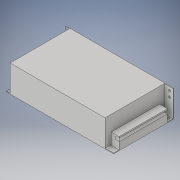
# Autodesk Inventor part: PowerS
Saved by Autodesk Inventor 2019.3 (Build 233278000, 278)
## iProperties
Created: 2020-08-28
Part Number: PowerS
Material: Generisch
Document SubType Name: Modeling
Designer: Nicolas Frick
Density: 1 g/cm^3
Appearance: Vorgabe
Author: Nicolas Frick
Autodesk Inventor part; units mm, degrees
ref_plane "YZ Plane" through (0, 0, 0) normal (1, 0, 0) x (0, 1, 0)
ref_plane "XZ Plane" through (0, 0, 0) normal (0, 1, 0) x (-1, 0, 0)
ref_plane "XY Plane" through (0, 0, 0) normal (0, 0, 1) x (1, 0, 0)
sketch "Skizze1" plane through (0, 0, 0) normal (0, 1, 0) x (-1, 0, 0)
  line L0 (88, 55) -> (-88, 55)
  line L1 (-88, 55) -> (-88, -55)
  line L2 (-88, -55) -> (88, -55)
  line L3 (88, -55) -> (88, 55)
  line L4 (88, 55) -> (-88, -55) construction
  line L5 (-88, 55) -> (88, -55) construction
  point P0 (0, 0)
  dimension "d0" = 176
  dimension "d1" = 110
  constraints: 12 end point, 2 midpoint, 2 parallel, 1 horizontal, 1 perpendicular
  measures "d0" distance of L2.end L1.end
  measures "d1" distance of L1.end L0.end
extrude "Extrusion1" add sketch "Skizze1" along normal blind 48.5
sketch "Skizze2" plane through (0, 0, 0) normal (0, -1, 0) x (1, 0, 0)
  line L0 (-88, 55) -> (88, 55) projected
  line L1 (-88, 55) -> (-95, 55)
  line L2 (-95, 55) -> (-95, -55.0669)
  line L3 (-95, -55.0669) -> (-88, -55.0669)
  line L4 (-88, -55.0669) -> (-88, -55)
  line L5 (88, 55) -> (104, 55)
  line L6 (104, 55) -> (104, -55.0669)
  line L7 (104, -55.0669) -> (88, -55.0669)
  line L8 (88, -55.0669) -> (88, -55)
  line L9 (-88, -55) -> (-88, 55) construction
  line L10 (88, 55) -> (88, -55) construction
  line L11 (-88, 55) -> (88, 55)
  line L12 (88, -55) -> (-88, -55)
  point P0 (0, 0)
  dimension "d4" = 7
  dimension "d5" = 16
  constraints: 20 end point, 5 parallel, 3 horizontal, 2 perpendicular, 2 point on line
  measures "d4" distance of L3.end L2.end
  measures "d5" distance of L6.end L7.end
extrude "Extrusion2" add sketch "Skizze2" along normal blind 1.3
sketch "Skizze3" plane through (88, 48.5, -55) normal (0, 0, -1) x (-1, 0, 0)
  line L0 (-16, -48.5) -> (183.0209, -48.5)
  line L1 (183.0209, -48.5) -> (183.0209, 0)
  line L2 (183.0209, 0) -> (-16, 0)
  line L3 (-16, 0) -> (-16, -48.5)
  point P0 (88, -48.5)
  constraints: 8 end point, 2 parallel, 1 horizontal, 1 perpendicular
extrude "Extrusion3" add sketch "Skizze3" along normal blind 1.3
sketch "Skizze4" plane through (0, 0, 0) normal (0, 1, 0) x (1, 0, 0)
  line L0 (104.0471, 54.3478) -> (104.0471, 44.3478) construction
  line L1 (104, 55.0669) -> (104, -55) construction
  line L2 (104, -55) -> (104, -45) construction
  line L3 (104, -45) -> (89.4287, -45)
  line L4 (89.4287, -45) -> (89.4287, 44.3478)
  line L5 (89.4287, 44.3478) -> (104, 44.3478)
  line L6 (104, 44.3478) -> (104, -45)
  point P0 (0, 0)
  dimension "d10" = 10
  dimension "d11" = 10
  constraints: 12 end point, 2 parallel, 1 horizontal, 1 perpendicular, 1 point on line, 1 vertical
  measures "d10" distance of L0.start L0.end
  measures "d11" distance of L1.end L2.end
extrude "Extrusion4" add sketch "Skizze4" along normal blind 21.5
sketch "Skizze5" plane through (104, -1.3, 55) normal (1, 0, 0) x (0, 0, -1)
  line L0 (99.3478, 1.3) -> (99.3478, 22.8) projected
  line L1 (99.3478, 14.5) -> (10.1519, 14.5)
  line L2 (10.1519, 14.5) -> (99.3478, 14.5)
  line L3 (99.3478, 14.5) -> (99.3478, 20.5)
  line L4 (99.3478, 20.5) -> (10.1519, 20.5)
  line L5 (10.1519, 20.5) -> (10.1519, 14.5)
  point P0 (55, 1.3)
  dimension "d15" = 6
  constraints: 10 end point, 2 parallel, 1 horizontal, 1 perpendicular, 1 point on line
  measures "d15" distance of L3.end L2.end
extrude "Extrusion5" cut sketch "Skizze5" against normal blind 6
sketch "Skizze6" plane through (88, 48.5, -56.3) normal (0, 0, -1) x (-1, 0, 0)
  line L0 (-16, 0) -> (-16, -48.5) projected
  line L1 (-7.8996, 0) -> (-7.8996, -24.25) construction
  line L2 (-16, -24.25) -> (4.0313, -24.25) construction
  line L3 (-16, -6.9035) -> (-9.4253, -6.9035) construction
  line L4 (-9.4253, -6.9035) -> (-9.4253, -17.0035) construction
  point P0 (88, -48.5)
  constraints: 8 end point, 3 coincident, 2 horizontal, 1 midpoint, 1 parallel, 1 point on line, 1 vertical
sketch "Skizze8" plane through (88, 48.5, -56.3) normal (0, 0, -1) x (-1, 0, 0)
  line L0 (182.9392, -17.1594) -> (180.3414, -17.1594) construction
  line L1 (180.3414, -0.3613) -> (180.3414, -6.3768) construction
  line L2 (180.3414, -0.3613) -> (180.3414, -26.3529) construction
  line L3 (183.0209, -48.5) -> (183.0209, 0) projected
  line L4 (183.0209, -40.3134) -> (162.5219, -40.3134) construction
  line L5 (162.5219, -0.3613) -> (162.5219, -37.3624) construction
  point P0 (88, -48.5)
  constraints: 10 end point, 3 coincident, 3 vertical, 2 horizontal, 1 point on line
hole "Bohrung3" at (-92.3414, 42.1232, -56.3) at (-92.3414, 22.1471, -56.3) at (-74.5219, 11.1376, -56.3) direction (0, 0, 1) diameter 3 end through all
sketch "Skizze9" plane through (88, 48.5, -56.3) normal (0, 0, -1) x (-1, 0, 0)
  circle A0 centre (180.3414, -6.3768) radius 1.5 projected
  arc A1 (180.3414, -4.6268) -> (180.3414, -8.1268) centre (180.3414, -6.3768) ccw
  arc A2 (180.3414, -24.6029) -> (180.3414, -28.1029) centre (180.3414, -26.3529) ccw
  line L0 (180.3414, -4.6268) -> (183.0209, -4.6268)
  line L1 (183.0209, -48.5) -> (183.0209, 0) projected
  line L2 (180.3414, -8.1268) -> (183.0209, -8.1268)
  line L3 (180.3414, -24.6029) -> (183.0209, -24.6029)
  line L4 (180.3414, -28.1029) -> (183.0209, -28.1029)
  line L5 (183.0209, -48.5) -> (183.0209, 0) projected
  point P0 (88, -48.5)
  dimension "d40" = 3.5
  dimension "d41" = 3.5
  constraints: 8 end point, 4 point on circle, 3 point on line, 2 centre point, 2 coincident, 2 horizontal, 2 tangent, 1 parallel, 1 perpendicular
  measures "d40" diameter of A1
  measures "d41" diameter of A2
extrude "Extrusion6" cut sketch "Skizze9" against normal blind 6
sketch "Skizze10" plane through (-88, 48.5, 55) normal (0, 0, 1) x (1, 0, 0)
  circle A0 centre (13.4781, -37.3624) radius 1.5 projected
  circle A1 centre (171.9687, -24.25) radius 1.5 projected
  point P0 (88, -48.5)
extrude "Extrusion7" add sketch "Skizze10" against normal blind 6
sketch "Skizze11" plane through (0, -1.3, 0) normal (0, -1, 0) x (1, 0, 0)
  line L0 (104.0362, -56.3543) -> (99.0362, -56.3543) construction
  line L1 (99.0362, -56.3543) -> (99.0362, -51.3543) construction
  line L2 (99.0362, -51.3543) -> (104.0362, -51.3543) construction
  line L3 (104.0362, -51.3543) -> (104.0362, -56.3543) construction
  point P0 (0, 0)
  dimension "d46" = 5
  dimension "d47" = 5
  constraints: 8 end point, 2 parallel, 1 coincident, 1 horizontal, 1 perpendicular
  measures "d46" distance of L1.end L2.end
  measures "d47" distance of L0.end L1.end
hole "Bohrung4" at (99.0362, -1.3, -51.3543) direction (0, 1, 0) diameter 4 end through all
hole "Bohrung5" at (97.4253, 41.5965, -56.3) at (97.4253, 31.4965, -56.3) at (83.9687, 24.25, -56.3) direction (0, 0, 1) diameter 3 end through all
sketch "Skizze13" plane through (88, 48.5, -56.3) normal (0, 0, -1) x (-1, 0, 0)
  circle A0 centre (-9.4253, -6.9035) radius 1.5 projected
  circle A1 centre (-9.4253, -17.0035) radius 1.5 projected
  point P0 (88, -48.5)
hole "Bohrung6" at (97.4253, 41.5965, -56.3) at (97.4253, 31.4965, -56.3) direction (0, 0, 1) diameter 4 end through all
sketch "Skizze14" plane through (-88, 48.5, 55) normal (0, 0, 1) x (1, 0, 0)
  circle A0 centre (171.9687, -24.25) radius 1.5 projected
  point P0 (88, -48.5)
extrude "Extrusion8" add sketch "Skizze14" against normal blind 6
